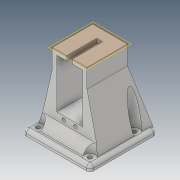
# Autodesk Inventor part: servoBracket
Saved by Autodesk Inventor 2018 (Build 220112000, 112)
## iProperties
Created: 2020-01-08
Part Number: servoBracket
Material: Generic
Document SubType Name: Modeling
Designer: anirudh
Density: 1 g/cm^3
Appearance: Default
Author: anirudh
Autodesk Inventor part; units mm, degrees
ref_plane "YZ Plane" through (0, 0, 0) normal (1, 0, 0) x (0, 1, 0)
ref_plane "XZ Plane" through (0, 0, 0) normal (0, 1, 0) x (-1, 0, 0)
ref_plane "XY Plane" through (0, 0, 0) normal (0, 0, 1) x (1, 0, 0)
sketch "Sketch1" plane through (0, 0, 0) normal (0, 0, 1) x (1, 0, 0)
  line L0 (0, 0) -> (22, 0)
  line L1 (22, 0) -> (22, 42)
  line L2 (0, 42) -> (0, 0)
  line L3 (-3.81, 0) -> (-3.81, 42)
  line L4 (-3.81, 42) -> (-3.81, 45.81)
  line L5 (25.81, 45.81) -> (25.81, 0)
  line L6 (25.81, 0) -> (25.81, -8)
  line L7 (25.81, -8) -> (-3.81, -8)
  line L8 (-3.81, -8) -> (-3.81, 0)
  line L9 (-3.81, 45.81) -> (8.5, 45.81)
  line L10 (8.5, 45.81) -> (8.5, 42)
  line L11 (0, 42) -> (8.5, 42)
  line L12 (13.5, 42) -> (22, 42)
  line L13 (13.5, 42) -> (13.5, 45.81)
  line L14 (13.5, 45.81) -> (25.81, 45.81)
  dimension "d1" = 22
  dimension "d11" = 5
  constraints: 30 end point, 4 perpendicular, 3 horizontal, 3 point on line, 1 vertical
  measures "d1" distance of L0.start L0.end
  measures "d11" distance of L10.end L12.start
extrude "Extrusion1" add sketch "Sketch1" along normal blind 30.7
sketch "Sketch3" plane through (0, 0, 0) normal (0, 0, -1) x (-1, 0, 0)
  line L0 (-25.81, 45.81) -> (-25.81, -8) projected
  line L1 (3.81, -8) -> (3.81, 45.81) projected
  line L2 (-25.81, 45.81) -> (3.81, 45.81)
  line L3 (3.81, 45.81) -> (3.81, -8)
  line L4 (3.81, -8) -> (-25.81, -8)
  line L5 (-25.81, -8) -> (-25.81, 45.81)
  point P0 (0, 0)
  constraints: 8 end point, 2 parallel, 1 horizontal, 1 perpendicular
extrude "Extrusion2" add sketch "Sketch3" along normal blind 3.81
sketch "Sketch4" plane through (0, 0, 0) normal (0, 0, 1) x (1, 0, 0)
  line L0 (8.5, 45.81) -> (8.5, 42) projected
  line L1 (13.5, 42) -> (13.5, 45.81) projected
  line L2 (8.5, 45.81) -> (13.5, 45.81)
  line L3 (13.5, 45.81) -> (13.5, 42)
  line L4 (13.5, 42) -> (8.5, 42)
  line L5 (8.5, 42) -> (8.5, 45.81)
  point P0 (0, 0)
  constraints: 8 end point, 2 parallel, 1 horizontal, 1 perpendicular
extrude "Extrusion3" add sketch "Sketch4" along normal blind 5
ref_plane "Work Plane1" through (-3.81, -19.8364, 30.7) normal (0, -1, 0) x (1, 0, 0)
sketch "Sketch5" plane through (-3.81, -19.8364, 30.7) normal (0, -1, 0) x (1, 0, 0)
  line L0 (0, 0) -> (0, -34.51) projected
  line L1 (25.81, 0) -> (3.81, 0) projected
  line L2 (14.81, 11.176) -> (43.385, 11.176)
  line L3 (43.385, 11.176) -> (43.385, -45.974)
  line L4 (43.385, -45.974) -> (-13.765, -45.974)
  line L5 (-13.765, -45.974) -> (-13.765, 11.176)
  line L6 (-13.765, 11.176) -> (14.81, 11.176)
  point P0 (3.81, -30.7)
  point P1 (29.62, 0)
  dimension "d20" = 28.575
  dimension "d22" = 57.15
  dimension "d23" = 57.15
  constraints: 10 end point, 3 perpendicular, 1 horizontal, 1 vertical
  measures "d20" distance of L2.start L2.end
  measures "d22" distance of L2.end L3.end
  measures "d23" distance of L3.end L4.end
extrude "Extrusion4" add sketch "Sketch5" against normal blind 5.08
sketch "Sketch6" plane through (-3.81, -8, 30.7) normal (0, -1, 0) x (1, 0, 0)
  line L0 (0, 0) -> (0, -34.51) projected
  line L1 (0, -34.51) -> (29.62, -34.51) projected
  line L2 (0, 0) -> (29.62, 0)
  line L3 (29.62, 0) -> (29.62, -34.51)
  line L4 (29.62, -34.51) -> (0, -34.51)
  line L5 (0, -34.51) -> (0, 0)
  point P0 (3.81, -30.7)
  constraints: 8 end point, 2 parallel, 1 horizontal, 1 perpendicular
extrude "Extrusion5" add sketch "Sketch6" along normal blind 7.62
chamfer "Chamfer1" distance 10.16 distance2 44.45 1 edges at (25.81, -14.7564, 13.445) measured on face at (26.31, -14.7564, 13.445)
chamfer "Chamfer2" distance 10.16 distance2 44.45 1 edges at (-3.81, -14.7564, 13.445) measured on face at (-4.31, -14.7564, 13.445)
chamfer "Chamfer3" distance 11.43 distance2 44.45 3 edges at (-8.89, -14.7564, -3.81) (11, -14.7564, -3.81) (30.89, -14.7564, -3.81) measured on face at (-8.89, -14.7564, -4.31) measured on face at (11, -14.7564, -4.31) measured on face at (30.89, -14.7564, -4.31)
ref_plane "Work Plane2" through (-3.81, 45.81, 30.7) normal (0, 1, 0) x (1, 0, 0)
sketch "Sketch7" plane through (-3.81, -19.8364, 30.7) normal (0, -1, 0) x (1, 0, 0)
  circle A0 centre (37.0114, -33.249) radius 1.8
  circle A1 centre (-7.3914, -33.249) radius 1.8
  point P0 (3.81, -30.7)
  point P1 (-10.16, -45.94)
  dimension "d48" = 3.6
  dimension "d49" = 3.6
  constraints: 2 centre point
  measures "d48" diameter of A0
  measures "d49" diameter of A1
extrude "Extrusion6" cut sketch "Sketch7" against normal blind 66.9925
sketch "Sketch9" plane through (-3.81, 45.81, 30.7) normal (0, 1, 0) x (1, 0, 0)
  circle A0 centre (37.0114, 33.249) radius 1.8 projected
  circle A1 centre (37.0114, 33.249) radius 4.445
  circle A2 centre (-7.3914, 33.249) radius 1.8 projected
  circle A3 centre (-7.3914, 33.249) radius 4.445
  point P0 (3.81, 30.7)
  dimension "d50" = 8.89
  dimension "d51" = 8.89
  constraints: 2 centre point, 2 coincident
  measures "d50" diameter of A1
  measures "d51" diameter of A3
extrude "Extrusion7" cut sketch "Sketch9" against normal blind 60.579 contours A0 | A1 | A2 | A3
sketch "Sketch10" plane through (0, 0, 30.7) normal (0, 0, 1) x (1, 0, 0)
  line L0 (22, 0) -> (22, 42) projected
  line L1 (22, 0) -> (0, 0) projected
  circle A0 centre (6, -3) radius 1.55
  circle A1 centre (16, -3) radius 1.55
  dimension "d57" = 3.1
  dimension "d58" = 3.1
  constraints: 2 centre point
  measures "d57" diameter of A0
  measures "d58" diameter of A1
extrude "Extrusion8" cut sketch "Sketch10" against normal blind 25.4
sketch "Sketch11" plane through (-3.81, -14.7564, 30.7) normal (0, 1, 0) x (1, 0, 0)
  circle A0 centre (-7.415, -4.826) radius 1.8
  circle A1 centre (37.035, -4.826) radius 1.8
  point P0 (3.81, 30.7)
  point P1 (-13.765, -11.176)
  point P2 (43.385, -11.176)
  dimension "d66" = 3.6
  constraints: 2 centre point
  measures "d66" diameter of A1
extrude "Extrusion9" cut sketch "Sketch11" against normal blind 25.4
chamfer "Chamfer4" distance 6.604 distance2 8.382 1 edges at (11, -14.7564, 30.7) measured on face at (11, -14.7564, 31.2)
sketch "Sketch12" plane through (-3.81, 45.81, 30.7) normal (0, 1, 0) x (1, 0, 0)
  circle A0 centre (-7.415, -4.826) radius 1.8 projected
  circle A1 centre (-7.415, -4.826) radius 4.445
  circle A2 centre (37.035, -4.826) radius 1.8 projected
  circle A3 centre (37.035, -4.826) radius 4.445
  point P0 (3.81, 30.7)
  dimension "d72" = 8.89
  dimension "d73" = 8.89
  constraints: 2 centre point, 2 coincident
  measures "d72" diameter of A1
  measures "d73" diameter of A3
extrude "Extrusion10" cut sketch "Sketch12" against normal blind 60.579 contours A0 | A1 | A2 | A3
fillet "Fillet1" radius 3.048 8 edges at (11, -14.7564, 41.876) (39.575, -14.7564, 13.301) (-17.575, -14.7564, 13.301) (11, -14.7564, -15.274) (39.575, -17.2964, 41.876) (-17.575, -17.2964, 41.876) (39.575, -17.2964, -15.274) (-17.575, -17.2964, -15.274)
body "Solid1"
